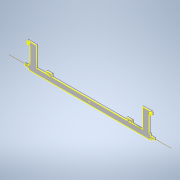
# Autodesk Inventor part: rod_2
Saved by Autodesk Inventor 2022 (Build 260153000, 153)
## iProperties
Created: 2023-04-07
Part Number: rod_2
Material: 一般
Document SubType Name: Modeling
Designer: may9c
Density: 79.16 g/cm^3
Appearance: 預設
Mass: 822.393 g
Surface Area: 88.4 cm^2
Volume: 10.389 cm^3
Author: may9c
Autodesk Inventor part; units mm, degrees
ref_plane "YZ Plane" through (0, 0, 0) normal (1, 0, 0) x (0, 1, 0)
ref_plane "XY Plane" through (0, 0, 0) normal (0, 0, 1) x (1, 0, 0)
sketch "草圖1" plane through (0, 0, 0) normal (0, 0, 1) x (1, 0, 0)
  line L0 (0, 6) -> (0, -6)
  line L1 (0, -6) -> (-139, -6)
  line L2 (-139, -6) -> (-139, 6)
  line L3 (-148, 2) -> (-139, 2)
  line L4 (-139, 2) -> (-139, -2)
  line L5 (-139, -2) -> (-148, -2)
  line L6 (-148, -2) -> (-148, 2)
  line L7 (-207.2, 0) -> (207.2, 0) projected
  line L8 (0, -9.6) -> (0, 15.6) projected
  line L9 (0, -6) -> (139, -6)
  line L10 (139, -6) -> (139, 6)
  line L11 (148, 2) -> (139, 2)
  line L12 (139, -2) -> (148, -2)
  line L13 (148, -2) -> (148, 2)
  line L14 (-148, -2) -> (-139, -2)
  line L15 (-139, -2) -> (-139, -6)
  line L16 (139, -6) -> (139, -2)
  line L17 (139, -2) -> (148, -2)
  line L18 (148, -2) -> (148, 2)
  line L19 (148, 2) -> (139, 2)
  line L20 (139, 2) -> (139, 6)
  line L21 (-139, 6) -> (-139, 2)
  line L22 (-139, 2) -> (-148, 2)
  line L23 (-148, 2) -> (-148, -2)
  line L24 (-97.5, 7) -> (-97.5, 12)
  line L25 (-97.5, 12) -> (-87.5, 12)
  line L26 (-90, 7) -> (-97.5, 7)
  line L27 (-90, 7) -> (-90, 5)
  line L28 (-90, 5) -> (-91, 5)
  line L29 (-91, 5) -> (-91, 6)
  line L30 (97.5, 7) -> (97.5, 12)
  line L31 (97.5, 12) -> (87.5, 12)
  line L32 (90, 7) -> (97.5, 7)
  line L33 (90, 7) -> (90, 5)
  line L34 (90, 5) -> (91, 5)
  line L35 (91, 5) -> (91, 6)
  line L36 (-139, 6) -> (-91, 6)
  line L37 (-85.5, 6) -> (85.5, 6)
  line L38 (91, 6) -> (139, 6)
  line L39 (-87.5, 12) -> (-85.5, 12)
  line L40 (-85.5, 12) -> (-85.5, 6)
  line L41 (87.5, 12) -> (85.5, 12)
  line L42 (85.5, 12) -> (85.5, 6)
  point P0 (0, 0)
  point P1 (-139, 2)
  dimension "d2" = 4
  dimension "d13" = 2
  dimension "d14" = 2
  dimension "d17" = 12
  constraints: 82 end point, 13 symmetric about line, 9 horizontal, 3 parallel, 3 perpendicular, 2 point on line, 1 collinear, 1 other
  measures "d2" distance between parallel lines of L5 L3
  measures "d13" distance of L25.end L39.end
  measures "d14" distance of L31.end L41.end
  measures "d17" distance between parallel lines of L1 L36
extrude "擠出1" add sketch "草圖1" along normal blind 3
ref_plane "工作平面1" through (0, 0, 1.5) normal (0, 0, 1) x (1, 0, 0)
sketch "草圖7" plane through (0, 0, 0) normal (0, 0, -1) x (-1, 0, 0)
  line L0 (-207.2, 0) -> (207.2, 0) projected
  circle A0 centre (132.5, 0) radius 12.5
  line L1 (148, -2) -> (139, -2) projected
  line L2 (145, -2) -> (145, 2)
  line L3 (139, 2) -> (148, 2) projected
  line L4 (148, 2) -> (148, -2) projected
  circle A1 centre (132.5, 0) radius 2.05
  point P0 (0, 0)
  dimension "d36" = 25
  dimension "d37" = 3
  dimension "d38" = 4.1
  constraints: 2 centre point, 2 end point, 2 point on line, 1 coincident, 1 tangent, 1 vertical
  measures "d36" diameter of A0
  measures "d37" distance between parallel lines of L4 L2
  measures "d38" diameter of A1
extrude "擠出5" cut sketch "草圖7" against normal up to surface (3 mm away) contours A1 L0 | L0 A1
sketch "草圖8" plane through (0, 0, 3) normal (0, 0, 1) x (1, 0, 0)
  line L0 (-91, 6) -> (-139, 6) projected
  line L1 (-136, 6) -> (-121, 6)
  line L2 (-121, 6) -> (-121, 51)
  line L3 (-121, 51) -> (-136, 51)
  line L4 (-136, 43) -> (-136, 6)
  line L5 (-139, 6) -> (-139, 2) projected
  line L6 (-136, 51) -> (-142.5, 51)
  line L7 (-142.5, 51) -> (-142.5, 43)
  line L8 (-142.5, 43) -> (-136, 43)
  circle A0 centre (-138.5, 47) radius 2.05
  circle A1 centre (-132.5, 0) radius 2.05 projected
  circle A2 centre (-138.5, 47) radius 6.5 construction
  line L9 (-139, 2) -> (-148, 2) projected
  line L10 (-148, 2) -> (-148, 58.0765) construction
  line L11 (-148, 58.0765) -> (-145, 58.0765) construction
  line L12 (-145, 58.0765) -> (-145, 42.2693) construction
  line L13 (-137.3204, 6) -> (-136, 6)
  line L14 (-136, 6) -> (-136, 16.271)
  circle A3 centre (-132.5, 16.6771) radius 2.05
  circle A4 centre (-132.5, 16.6771) radius 12.5 construction
  point P0 (0, 0)
  dimension "d55" = 25
  dimension "d41" = 3
  dimension "d42" = 15
  dimension "d43" = 45
  dimension "d45" = 8
  dimension "d49" = 3
  dimension "d50" = 13
  dimension "d51" = 47
  dimension "d52" = 6.5
  constraints: 24 end point, 5 perpendicular, 3 centre point, 3 horizontal, 3 parallel, 3 point on line, 2 coincident, 2 equal radius, 1 tangent, 1 vertical, 1 vertical alignment, 3 other
  measures "d41" distance between parallel lines of L5 L4
  measures "d42" distance of L2.end L3.end
  measures "d43" distance between parallel lines of L0 L3
  measures "d45" distance between parallel lines of L8 L6
  measures "d49" distance between parallel lines of L10 L12
  measures "d50" diameter of A2
  measures "d51" vertical distance of A1.centre A0.centre
  measures "d52" distance between parallel lines of L4 L7
extrude "擠出6" add sketch "草圖8" against normal up to surface (3 mm away) contours L0 L4 L8 L7 L6 L3 L2 | A1 | A3
fillet "圓角2" radius 2 2 edges at (-142.5, 51, 1.5) (-142.5, 43, 1.5)
mirror "鏡射6" about plane through (0, 0, 0) normal (1, 0, 0) of "擠出5", "擠出6", "圓角2"
sketch "草圖9" plane through (0, 0, 3) normal (0, 0, 1) x (1, 0, 0)
  arc A0 (140.5, 43) -> (142.5, 45) centre (140.5, 45) ccw projected
  line L0 (142.5, 49) -> (142.5, 45) projected
  arc A1 (142.5, 49) -> (140.5, 51) centre (140.5, 49) ccw projected
  line L1 (121, 51) -> (140.5, 51) projected
  line L2 (121, 6) -> (121, 51) projected
  line L3 (121, 6) -> (91, 6) projected
  line L4 (91, 6) -> (91, 5) projected
  line L5 (91, 5) -> (90, 5) projected
  line L6 (90, 5) -> (90, 7) projected
  line L7 (90, 7) -> (97.5, 7) projected
  line L8 (97.5, 7) -> (97.5, 12) projected
  line L9 (97.5, 12) -> (85.5, 12) projected
  line L10 (85.5, 12) -> (85.5, 6) projected
  line L11 (85.5, 6) -> (-85.5, 6) projected
  line L12 (-85.5, 6) -> (-85.5, 12) projected
  line L13 (-85.5, 12) -> (-97.5, 12) projected
  line L14 (-97.5, 12) -> (-97.5, 7) projected
  line L15 (-97.5, 7) -> (-90, 7) projected
  line L16 (-90, 7) -> (-90, 5) projected
  line L17 (-90, 5) -> (-91, 5) projected
  line L18 (-91, 5) -> (-91, 6) projected
  line L19 (-91, 6) -> (-121, 6) projected
  line L20 (-121, 6) -> (-121, 51) projected
  line L21 (-121, 51) -> (-140.5, 51) projected
  arc A2 (-140.5, 51) -> (-142.5, 49) centre (-140.5, 49) ccw projected
  line L22 (-142.5, 49) -> (-142.5, 45) projected
  arc A3 (-142.5, 45) -> (-140.5, 43) centre (-140.5, 45) ccw projected
  line L23 (-140.5, 43) -> (-136, 43) projected
  line L24 (-136, 43) -> (-136, 6) projected
  line L25 (-136, 6) -> (-139, 6) projected
  line L26 (-139, 6) -> (-139, 2) projected
  line L27 (-139, 2) -> (-148, 2) projected
  line L28 (-148, 2) -> (-148, -2) projected
  line L29 (-148, -2) -> (-139, -2) projected
  line L30 (-139, -2) -> (-139, -6) projected
  line L31 (-139, -6) -> (139, -6) projected
  line L32 (139, -6) -> (139, -2) projected
  line L33 (139, -2) -> (148, -2) projected
  line L34 (148, -2) -> (148, 2) projected
  line L35 (148, 2) -> (139, 2) projected
  line L36 (139, 2) -> (139, 6) projected
  line L37 (139, 6) -> (136, 6) projected
  line L38 (136, 43) -> (136, 6) projected
  line L39 (140.5, 43) -> (136, 43) projected
  circle A4 centre (138.5, 47) radius 2.05 projected
  circle A5 centre (-138.5, 47) radius 2.05 projected
  point P0 (0, 0)
